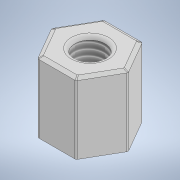
# Autodesk Inventor part: ASL-306KE
Saved by Autodesk Inventor 2022 (Build 260153000, 153)
## iProperties
Created: 2022-03-25
Part Number: ASL-306KE
Material: 一般
Document SubType Name: Modeling
Designer: masayuki
Density: 1 g/cm^3
Appearance: 既定
Author: masayuki
Autodesk Inventor part; units mm, degrees
ref_plane "YZ Plane" through (0, 0, 0) normal (1, 0, 0) x (0, 1, 0)
ref_plane "XZ Plane" through (0, 0, 0) normal (0, 1, 0) x (-1, 0, 0)
ref_plane "XY Plane" through (0, 0, 0) normal (0, 0, 1) x (1, 0, 0)
sketch "スケッチ1" plane through (0, 0, 0) normal (0, 1, 0) x (-1, 0, 0)
  line L0 (-3.1754, 0) -> (-1.5877, 2.75)
  line L1 (-1.5877, 2.75) -> (1.5877, 2.75)
  line L2 (1.5877, 2.75) -> (3.1754, 0)
  line L3 (3.1754, 0) -> (1.5877, -2.75)
  line L4 (1.5877, -2.75) -> (-1.5877, -2.75)
  line L5 (-1.5877, -2.75) -> (-3.1754, 0)
  point P0 (0, 0)
  point P1 (0, 0)
  dimension "d0" = 5.5
  constraints: 12 end point, 1 coincident, 13 other
  measures "d0" distance between parallel lines of L4 L1
extrude "押し出し1" add sketch "スケッチ1" along normal blind 6
sketch "スケッチ2" plane through (0, 6, 0) normal (0, 1, 0) x (1, 0, 0)
  circle A0 centre (0, 0) radius 1.25
  dimension "d3" = 2.5
  constraints: 1 centre point, 1 coincident
  measures "d3" diameter of A0
extrude "押し出し2" cut sketch "スケッチ2" against normal through all
thread "ねじ1" size "M3x0.5" class "6H" standard "ISO Metric profile" full length
chamfer "面取り1" distance 0.3 angle 30 6 edges at (2.3816, 6, -1.375) (2.3816, 6, 1.375) (0, 6, 2.75) (-2.3816, 6, 1.375) (-2.3816, 6, -1.375) (0, 6, -2.75) measured on face at (0.0502, 6, 2.247)
chamfer "面取り2" distance 0.3 angle 30 6 edges at (-2.3816, 0, -1.375) (-2.3816, 0, 1.375) (0, 0, -2.75) (2.3816, 0, -1.375) (2.3816, 0, 1.375) (0, 0, 2.75) measured on face at (0.0502, 0, 2.247)
fillet "フィレット1" radius 0.3 2 edges at (-1.25, 0, 0) (-1.25, 6, 0)
fillet "フィレット3" radius 0.2 18 edges at (-3.0022, 5.9134, 0) (-3.0022, 0.0866, 0) (-3.1754, 3, 0) (-1.5011, 5.9134, -2.6) (-1.5011, 0.0866, -2.6) (-1.5877, 3, -2.75) (1.5011, 5.9134, -2.6) (1.5011, 0.0866, -2.6) (1.5877, 3, -2.75) (3.0022, 5.9134, 0) (3.0022, 0.0866, 0) (3.1754, 3, 0) (1.5011, 5.9134, 2.6) (1.5011, 0.0866, 2.6) (1.5877, 3, 2.75) (-1.5011, 5.9134, 2.6) (-1.5011, 0.0866, 2.6) (-1.5877, 3, 2.75)
